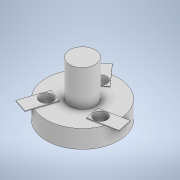
# Autodesk Inventor part: hand_shaft
Saved by Autodesk Inventor 2021 (Build 250183000, 183)
## iProperties
Created: 2021-11-07
Part Number: hand_shaft
Material: Generic
Document SubType Name: Modeling
Designer: shubh
Density: 1 g/cm^3
Appearance: Default
Author: shubh
Autodesk Inventor part; units mm, degrees
ref_plane "YZ Plane" through (0, 0, 0) normal (1, 0, 0) x (0, 1, 0)
ref_plane "XZ Plane" through (0, 0, 0) normal (0, 1, 0) x (-1, 0, 0)
ref_plane "XY Plane" through (0, 0, 0) normal (0, 0, 1) x (1, 0, 0)
sketch "Sketch1" plane through (0, 0, 0) normal (0, 1, 0) x (-1, 0, 0)
  circle A0 centre (0, 0) radius 12.7
  dimension "d0" = 25.4
  constraints: 1 centre point, 1 coincident
  measures "d0" diameter of A0
extrude "Extrusion1" add sketch "Sketch1" along normal blind 6.35
sketch "Sketch2" plane through (0, 6.35, 0) normal (0, 1, 0) x (1, 0, 0)
  line L0 (0, 0) -> (-6.35, 0)
  circle A0 centre (-6.35, -6.35) radius 2.2451
  line L1 (-3.175, -4.7625) -> (-7.9375, -3.175)
  line L2 (-7.9375, -3.175) -> (-11.0117, -12.3975)
  line L3 (-3.175, -4.7625) -> (-6.2492, -13.985)
  line L4 (-11.0117, -12.3975) -> (-6.2492, -13.985)
  circle A1 centre (8.6743, -2.3243) radius 2.2451
  line L5 (6.7184, -5.2866) -> (16.2423, -3.3376)
  line L6 (16.2423, -3.3376) -> (15.2359, 1.5806)
  line L7 (5.7119, -0.3684) -> (15.2359, 1.5806)
  line L8 (5.7119, -0.3684) -> (6.7184, -5.2866)
  circle A2 centre (-2.3243, 8.6743) radius 2.2451
  line L9 (1.2191, 8.4616) -> (-5.2307, 15.7351)
  line L10 (-5.2307, 15.7351) -> (-8.9867, 12.4044)
  line L11 (-2.5369, 5.1309) -> (-8.9867, 12.4044)
  line L12 (-2.5369, 5.1309) -> (1.2191, 8.4616)
  dimension "d5" = 360
  constraints: 26 end point, 3 centre point, 3 perpendicular, 1 horizontal, 31 other
extrude "Extrusion2" add sketch "Sketch2" along normal blind 0.254
sketch "Sketch3" plane through (-6.35, 6.35, 6.35) normal (0, 1, 0) x (1, 0, 0)
  point P0 (6.35, 6.35)
sketch "Sketch4" plane through (0, 6.35, 0) normal (0, 1, 0) x (1, 0, 0)
  circle A0 centre (-6.35, -6.35) radius 2.2451
  circle A1 centre (8.6743, -2.3243) radius 2.2451
  circle A2 centre (-2.3243, 8.6743) radius 2.2451
  point P0 (0, 0)
  dimension "d11" = 360
  constraints: 3 centre point, 7 other
extrude "Extrusion3" cut sketch "Sketch4" against normal blind 12.7
sketch "Sketch5" plane through (0, 6.35, 0) normal (0, 1, 0) x (1, 0, 0)
  circle A0 centre (0, 0) radius 4.4901
  constraints: 1 centre point, 1 coincident
extrude "Extrusion4" add sketch "Sketch5" along normal blind 12.7
body "Solid1"
